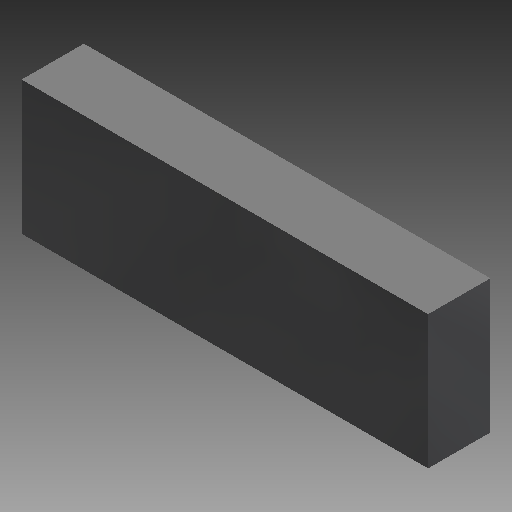
# Autodesk Inventor part: LiFePo
Saved by Autodesk Inventor 2018.3 (Build 223284000, 284)
## iProperties
Created: 2016-10-17
Part Number: LiFePo
Material: 一般
Document SubType Name: Modeling
Designer: Shinichi
Density: 1 g/cm^3
Appearance: 既定
Author: Shinichi
Autodesk Inventor part; units mm, degrees
ref_plane "YZ Plane" through (0, 0, 0) normal (1, 0, 0) x (0, 1, 0)
ref_plane "XZ Plane" through (0, 0, 0) normal (0, 1, 0) x (-1, 0, 0)
ref_plane "XY Plane" through (0, 0, 0) normal (0, 0, 1) x (1, 0, 0)
sketch "スケッチ1" plane through (0, 0, 0) normal (0, 0, 1) x (1, 0, 0)
  line L0 (-68.5, -22.5) -> (68.5, -22.5)
  line L1 (68.5, -22.5) -> (68.5, 22.5)
  line L2 (68.5, 22.5) -> (-68.5, 22.5)
  line L3 (-68.5, 22.5) -> (-68.5, -22.5)
  line L4 (-68.5, -22.5) -> (68.5, 22.5) construction
  line L5 (68.5, -22.5) -> (-68.5, 22.5) construction
  point P0 (0, 0)
  dimension "d0" = 137
  dimension "d1" = 45
  constraints: 12 end point, 2 midpoint, 2 parallel, 1 horizontal, 1 perpendicular
  measures "d0" distance of L2.end L1.end
  measures "d1" distance of L1.end L0.end
extrude "押し出し1" add sketch "スケッチ1" along normal blind 21
